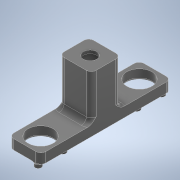
# Autodesk Inventor part: PotHolder
Saved by Autodesk Inventor 2022 (Build 260153000, 153)
## iProperties
Created: 2021-11-22
Part Number: PotHolder
Material: Genérico
Document SubType Name: Modeling
Designer: JK
Density: 1 g/cm^3
Appearance: Suave - Negro
Author: JK
Autodesk Inventor part; units mm, degrees
ref_plane "YZ Plane" through (0, 0, 0) normal (1, 0, 0) x (0, 1, 0)
ref_plane "XZ Plane" through (0, 0, 0) normal (0, 1, 0) x (-1, 0, 0)
ref_plane "XY Plane" through (0, 0, 0) normal (0, 0, 1) x (1, 0, 0)
sketch "Boceto7" plane through (0, 0, 0) normal (0, 1, 0) x (-1, 0, 0)
  line L0 (-6.5, 12.2) -> (6.5, 12.2)
  line L1 (6.5, 12.2) -> (6.5, -12.2)
  line L2 (6.5, -12.2) -> (-6.5, -12.2)
  line L3 (-6.5, -12.2) -> (-6.5, 12.2)
  line L4 (-6.5, 12.2) -> (6.5, -12.2) construction
  line L5 (6.5, 12.2) -> (-6.5, -12.2) construction
  line L6 (6.5, 12.2) -> (-6.5, 12.2)
  line L7 (-6.5, 12.2) -> (-6.5, 26.4)
  line L8 (-6.5, 26.4) -> (6.5, 26.4)
  line L9 (6.5, 26.4) -> (6.5, 12.2)
  line L10 (6.5, -12.2) -> (-6.5, -12.2)
  line L11 (-6.5, -12.2) -> (-6.5, -26.4)
  line L12 (-6.5, -26.4) -> (6.5, -26.4)
  line L13 (6.5, -26.4) -> (6.5, -12.2)
  line L14 (4.8, 24.8) -> (-4.8, 24.8)
  line L15 (-4.8, 24.8) -> (-4.8, 15.2)
  line L16 (-4.8, 15.2) -> (4.8, 15.2)
  line L17 (4.8, 15.2) -> (4.8, 24.8)
  line L18 (4.8, -15.2) -> (-4.8, -15.2)
  line L19 (-4.8, -15.2) -> (-4.8, -24.8)
  line L20 (-4.8, -24.8) -> (4.8, -24.8)
  line L21 (4.8, -24.8) -> (4.8, -15.2)
  line L22 (-4.8, 24.8) -> (4.8, 24.8)
  line L23 (4.8, 24.8) -> (4.8, 15.2)
  line L24 (4.8, 15.2) -> (-4.8, 15.2)
  line L25 (-4.8, 15.2) -> (-4.8, 24.8)
  line L26 (-4.8, 24.8) -> (4.8, 15.2) construction
  line L27 (4.8, 24.8) -> (-4.8, 15.2) construction
  line L28 (-4.8, -15.2) -> (4.8, -15.2)
  line L29 (4.8, -15.2) -> (4.8, -24.8)
  line L30 (4.8, -24.8) -> (-4.8, -24.8)
  line L31 (-4.8, -24.8) -> (-4.8, -15.2)
  line L32 (-4.8, -15.2) -> (4.8, -24.8) construction
  line L33 (4.8, -15.2) -> (-4.8, -24.8) construction
  point P0 (0, 0)
  point P1 (-6.5, 12.2)
  point P2 (0, 20)
  point P3 (0, -20)
  point P4 (0, -20)
  point P5 (0, 0)
  dimension "d23" = 9.6
  dimension "d24" = 9.6
  dimension "d26" = 1.6
  dimension "d28" = 3
  dimension "d30" = 1.6
  dimension "d31" = 3
  dimension "d43" = 40
  dimension "d48" = 13
  constraints: 68 end point, 14 parallel, 8 midpoint, 7 horizontal, 7 perpendicular, 6 collinear, 2 equal length, 1 point on line, 1 vertical alignment
  measures "d23" distance of L16.end L14.start
  measures "d24" distance of L15.end L16.end
  measures "d26" distance between parallel lines of L14 L8
  measures "d28" distance between parallel lines of L0 L16
  measures "d30" distance between parallel lines of L12 L20
  measures "d31" distance between parallel lines of L2 L18
  measures "d43" distance of point (0, -20) point (0, 20)
  measures "d48" distance between parallel lines of L7 L9
extrude "Extrusión4" add sketch "Boceto7" along normal blind 4
sketch "Boceto8" plane through (0, 4, 0) normal (0, 1, 0) x (1, 0, 0)
  circle A0 centre (0, -4.8061) radius 1.7
  circle A1 centre (0, 5.1939) radius 1.7
  point P0 (0, 0.1939)
  dimension "d35" = 3.4
  dimension "d49" = 5
  dimension "d50" = 5
  constraints: 2 centre point, 2 vertical alignment, 1 equal radius
  measures "d35" diameter of A0
  measures "d49" distance of A0.centre point (0, 0.194)
  measures "d50" distance of point (0, 0.194) A1.centre
fillet "Empalme3" radius 2 4 edges at (-6.5, 2, 26.4) (6.5, 2, 26.4) (-6.5, 2, -26.4) (6.5, 2, -26.4)
sketch "Boceto9" plane through (0, 4, 0) normal (0, 1, 0) x (1, 0, 0)
  line L0 (-6.5, 24.4) -> (-6.5, -24.4) projected
  line L1 (6.5, -6) -> (-6.5, -6)
  line L2 (-6.5, -6) -> (-6.5, 6)
  line L3 (-6.5, 6) -> (6.5, 6)
  line L4 (6.5, 6) -> (6.5, -6)
  line L5 (6.5, -6) -> (-6.5, 6) construction
  line L6 (-6.5, -6) -> (6.5, 6) construction
  arc A0 (6.5, 24.4) -> (4.5, 26.4) centre (4.5, 24.4) ccw projected
  line L7 (4.5, 26.4) -> (-4.5, 26.4) projected
  arc A1 (-4.5, 26.4) -> (-6.5, 24.4) centre (-4.5, 24.4) ccw projected
  line L8 (-6.5, 24.4) -> (-6.5, -24.4) projected
  arc A2 (-6.5, -24.4) -> (-4.5, -26.4) centre (-4.5, -24.4) ccw projected
  line L9 (-4.5, -26.4) -> (4.5, -26.4) projected
  arc A3 (4.5, -26.4) -> (6.5, -24.4) centre (4.5, -24.4) ccw projected
  line L10 (6.5, -24.4) -> (6.5, 24.4) projected
  line L11 (-4.8, -24.8) -> (-4.8, -15.2) projected
  line L12 (-4.8, -15.2) -> (4.8, -15.2) projected
  line L13 (4.8, -15.2) -> (4.8, -24.8) projected
  line L14 (4.8, -24.8) -> (-4.8, -24.8) projected
  line L15 (-4.8, 15.2) -> (-4.8, 24.8) projected
  line L16 (-4.8, 24.8) -> (4.8, 24.8) projected
  line L17 (4.8, 24.8) -> (4.8, 15.2) projected
  line L18 (4.8, 15.2) -> (-4.8, 15.2) projected
  point P0 (0, 0)
  dimension "d44" = 12
  constraints: 12 end point, 2 midpoint, 2 parallel, 1 horizontal, 1 perpendicular, 1 point on line
  measures "d44" distance between parallel lines of L3 L1
extrude "Extrusión6" add sketch "Boceto9" along normal blind 18.3 contours L3 L4 L1 L0
fillet "Empalme4" radius 2 6 edges at (6.5, 13.15, 6) (6.5, 13.15, -6) (-6.5, 13.15, -6) (-6.5, 13.15, 6) (0, 4, -6) (0, 4, 6)
sketch "Boceto11" plane through (0, 0, 0) normal (0, -1, 0) x (1, 0, 0)
  circle A0 centre (0, 20) radius 5.1
  line L0 (-4.8, 15.2) -> (4.8, 15.2) projected
  line L1 (-4.8, 24.8) -> (4.8, 24.8)
  line L2 (4.8, 24.8) -> (4.8, 15.2)
  line L3 (4.8, 15.2) -> (-4.8, 15.2)
  line L4 (-4.8, 15.2) -> (-4.8, 24.8)
  line L5 (-4.8, 24.8) -> (4.8, 15.2) construction
  line L6 (4.8, 24.8) -> (-4.8, 15.2) construction
  line L7 (4.8, -24.8) -> (4.8, -15.2) projected
  line L8 (-4.8, -15.2) -> (4.8, -15.2)
  line L9 (4.8, -15.2) -> (4.8, -24.8)
  line L10 (4.8, -24.8) -> (-4.8, -24.8)
  line L11 (-4.8, -24.8) -> (-4.8, -15.2)
  line L12 (-4.8, -15.2) -> (4.8, -24.8) construction
  line L13 (4.8, -15.2) -> (-4.8, -24.8) construction
  circle A1 centre (0, -20) radius 5.1
  point P0 (0, 0)
  point P1 (0, 20)
  point P2 (0, 20)
  dimension "d54" = 10.2
  dimension "d55" = 10.2
  constraints: 24 end point, 5 midpoint, 4 parallel, 2 centre point, 2 coincident, 2 horizontal, 2 perpendicular
  measures "d54" diameter of A0
  measures "d55" diameter of A1
extrude "Extrusión8" cut sketch "Boceto11" against normal through all contours A0 L2 | L2 A0 L0 L4 L1 | L1 A0 | A0 L0 | L4 A0 | A1 L10 L11 L8 L7 | L7 A1 | A1 L10 | L8 A1 | A1 L11
sketch "Boceto12" plane through (0, 0, 0) normal (0, -1, 0) x (1, 0, 0)
  arc A0 (4.8, 18.2766) -> (4.8, 21.7234) centre (0, 20) ccw projected
  circle A1 centre (0, 20) radius 5.1
  arc A2 (4.8, -21.7234) -> (4.8, -18.2766) centre (0, -20) ccw projected
  circle A3 centre (0, -20) radius 5.1
  arc A4 (1.7234, -15.2) -> (-1.7234, -15.2) centre (0, -20) ccw projected
  line L0 (4.8, -15.2) -> (1.7234, -15.2) projected
  line L1 (4.8, -18.2766) -> (4.8, -15.2) projected
  arc A5 (4.8, -21.7234) -> (4.8, -18.2766) centre (0, -20) ccw projected
  line L2 (4.8, -24.8) -> (4.8, -21.7234) projected
  line L3 (1.7234, -24.8) -> (4.8, -24.8) projected
  arc A6 (-1.7234, -24.8) -> (1.7234, -24.8) centre (0, -20) ccw projected
  line L4 (-4.8, -24.8) -> (-1.7234, -24.8) projected
  line L5 (-4.8, -21.7234) -> (-4.8, -24.8) projected
  arc A7 (-4.8, -18.2766) -> (-4.8, -21.7234) centre (0, -20) ccw projected
  line L6 (-4.8, -15.2) -> (-4.8, -18.2766) projected
  line L7 (-1.7234, -15.2) -> (-4.8, -15.2) projected
  arc A8 (1.7234, 24.8) -> (-1.7234, 24.8) centre (0, 20) ccw projected
  line L8 (4.8, 24.8) -> (1.7234, 24.8) projected
  line L9 (4.8, 21.7234) -> (4.8, 24.8) projected
  arc A9 (4.8, 18.2766) -> (4.8, 21.7234) centre (0, 20) ccw projected
  line L10 (4.8, 15.2) -> (4.8, 18.2766) projected
  line L11 (1.7234, 15.2) -> (4.8, 15.2) projected
  arc A10 (-1.7234, 15.2) -> (1.7234, 15.2) centre (0, 20) ccw projected
  line L12 (-4.8, 15.2) -> (-1.7234, 15.2) projected
  line L13 (-4.8, 18.2766) -> (-4.8, 15.2) projected
  arc A11 (-4.8, 21.7234) -> (-4.8, 18.2766) centre (0, 20) ccw projected
  line L14 (-4.8, 24.8) -> (-4.8, 21.7234) projected
  line L15 (-1.7234, 24.8) -> (-4.8, 24.8) projected
  arc A12 (4.5, -26.4) -> (6.5, -24.4) centre (4.5, -24.4) ccw projected
  line L16 (6.5, 24.4) -> (6.5, -24.4) projected
  arc A13 (6.5, 24.4) -> (4.5, 26.4) centre (4.5, 24.4) ccw projected
  line L17 (-4.5, 26.4) -> (4.5, 26.4) projected
  arc A14 (-4.5, 26.4) -> (-6.5, 24.4) centre (-4.5, 24.4) ccw projected
  line L18 (-6.5, -24.4) -> (-6.5, 24.4) projected
  arc A15 (-6.5, -24.4) -> (-4.5, -26.4) centre (-4.5, -24.4) ccw projected
  line L19 (4.5, -26.4) -> (-4.5, -26.4) projected
  point P0 (0, 0)
  point P1 (-1.7234, 24.8)
  point P2 (-4.8, 21.7234)
  point P3 (1.7234, 24.8)
  point P4 (4.8, 18.2766)
  point P5 (-1.7234, 15.2)
  point P6 (-1.7234, -15.2)
  point P7 (-4.8, -18.2766)
  point P8 (-1.7234, -24.8)
  point P9 (4.8, -21.7234)
  point P10 (1.7234, -15.2)
  constraints: 2 centre point, 2 coincident
extrude "Extrusión9" add sketch "Boceto12" against normal up to surface (4 mm away) contours L10 L11 A1 | A1 L8 L9 | L12 L13 A1 | A1 L14 L15 | L2 L3 A3 | A3 L0 L1 | L4 L5 A3 | A3 L6 L7
fillet "Empalme5" radius 0.75 16 edges at (-5.1, 0, 20) (0, 0, 14.9) (5.1, 0, 20) (0, 0, 25.1) (-3.6062, 0, 23.6062) (-3.6062, 0, 16.3938) (3.6062, 0, 16.3938) (3.6062, 0, 23.6062) (-5.1, 0, -20) (0, 0, -25.1) (5.1, 0, -20) (0, 0, -14.9) (-3.6062, 0, -16.3938) (-3.6062, 0, -23.6062) (3.6062, 0, -23.6062) (3.6062, 0, -16.3938)
sketch "Boceto14" plane through (0, 0, 0) normal (0, -1, 0) x (1, 0, 0)
  circle A0 centre (0, 20) radius 5.85 projected
  arc A1 (6.5, -24.4) -> (4.5, -26.4) centre (4.5, -24.4) ccw projected
  line L0 (6.5, 24.4) -> (6.5, -24.4) projected
  arc A2 (4.5, 26.4) -> (6.5, 24.4) centre (4.5, 24.4) ccw projected
  line L1 (-4.5, 26.4) -> (4.5, 26.4) projected
  arc A3 (-6.5, 24.4) -> (-4.5, 26.4) centre (-4.5, 24.4) ccw projected
  line L2 (-6.5, -24.4) -> (-6.5, 24.4) projected
  arc A4 (-4.5, -26.4) -> (-6.5, -24.4) centre (-4.5, -24.4) ccw projected
  line L3 (4.5, -26.4) -> (-4.5, -26.4) projected
  circle A5 centre (0, -20) radius 5.1531
  circle A6 centre (4, -25) radius 1.25
  circle A7 centre (4, -15) radius 1.25
  point P0 (0, 0)
  dimension "d65" = 2.5
  dimension "d66" = 4
  dimension "d72" = 5
  dimension "d73" = 5
  constraints: 8 centre point, 1 equal radius, 1 tangent, 1 vertical alignment
  measures "d65" diameter of A7
  measures "d66" horizontal distance of A5.centre A7.centre
  measures "d72" vertical distance of A7.centre A5.centre
  measures "d73" vertical distance of A6.centre A5.centre
extrude "Extrusión11" add sketch "Boceto14" along normal blind 2 and the other way blind 1 contours A7 | A6 A1 | A1 A6
mirror "Simetría1" about plane through (0, 0, 0) normal (0, 0, 1) of "Extrusión11"
fillet "Empalme7" radius 0.75 16 edges at (3.6813, 0.2573, 16.2087) (2.7913, 0.1153, 15.3185) (5.0236, 0, 15.7175) (4.0791, 0, 13.7525) (2.7913, 0.1153, 24.6815) (3.6813, 0.2573, 23.7913) (4.0791, 0, 26.2475) (5.0236, 0, 24.2825) (2.7913, 0.1153, -15.3185) (3.6813, 0.2573, -16.2087) (4.0791, 0, -13.7525) (5.0236, 0, -15.7175) (2.7913, 0.1153, -24.6815) (3.6813, 0.2573, -23.7913) (4.0791, 0, -26.2475) (5.0236, 0, -24.2825)
sketch "Boceto16" plane through (0, 22.3, 0) normal (0, 1, 0) x (1, 0, 0)
  circle A0 centre (0, 0) radius 2.7
  dimension "d77" = 5.4
  constraints: 1 centre point, 1 coincident
  measures "d77" diameter of A0
extrude "Extrusión13" cut sketch "Boceto16" against normal through all
sketch "Boceto17" plane through (0, 0, 0) normal (0, -1, 0) x (1, 0, 0)
  circle A0 centre (0, 0) radius 4.6
  dimension "d80" = 9.2
  constraints: 1 centre point, 1 coincident
  measures "d80" diameter of A0
extrude "Extrusión14" cut sketch "Boceto17" against normal blind 21
fillet "Empalme8" radius 1 1 edges at (-4.6, 0, 0)
sketch "Boceto15" plane through (0, 0, 0) normal (0, -1, 0) x (1, 0, 0)
  line L0 (6.5, 24.4) -> (6.5, -24.4) projected
  line L1 (-6.5, 29.6309) -> (6.5, 29.6309)
  line L2 (6.5, 29.6309) -> (6.5, 10.3691)
  line L3 (6.5, 10.3691) -> (-6.5, 10.3691)
  line L4 (-6.5, 10.3691) -> (-6.5, 29.6309)
  arc A0 (4.891, 16.7906) -> (4.891, 23.2094) centre (0, 20) ccw projected
  line L5 (-6.5, 29.6309) -> (6.5, 10.3691) construction
  line L6 (6.5, 29.6309) -> (-6.5, 10.3691) construction
  line L7 (13.0536, 10.3534) -> (-14.653, 10.3534)
  line L8 (-14.653, 10.3534) -> (-14.653, -30.0958)
  line L9 (-14.653, -30.0958) -> (13.0536, -30.0958)
  line L10 (13.0536, -30.0958) -> (13.0536, 10.3534)
  point P0 (0, 0)
  point P1 (3.6743, 15.4478)
  point P2 (3.6743, 24.5522)
  point P3 (8, 10.3534)
  point P4 (-8, 10.3534)
  constraints: 20 end point, 4 parallel, 2 horizontal, 2 midpoint, 2 perpendicular, 1 point on line
sketch "Boceto10" plane through (0, 0, 0) normal (0, -1, 0) x (1, 0, 0)
  line L0 (8, 25.8) -> (8, 10.3534) projected
  arc A0 (8, 25.8) -> (6, 27.8) centre (6, 25.8) ccw projected
  line L1 (-6, 27.8) -> (6, 27.8) projected
  arc A1 (-6, 27.8) -> (-8, 25.8) centre (-6, 25.8) ccw projected
  line L2 (-8, 10.3534) -> (-8, 25.8) projected
  line L3 (-4.8, 15.2) -> (4.8, 15.2) projected
  line L4 (-2.4608, 24.8) -> (2.8, 24.8)
  line L5 (2.8, 24.8) -> (2.8, 15.2)
  line L6 (2.8, 15.2) -> (-2.4608, 15.2)
  line L7 (-2.4608, 15.2) -> (-2.4608, 24.8)
  line L8 (-2.4608, 24.8) -> (2.8, 15.2) construction
  line L9 (2.8, 24.8) -> (-2.4608, 15.2) construction
  line L10 (-4.8, -24.8) -> (4.8, -24.8) projected
  line L11 (-2.6635, -15.2) -> (2.8, -15.2)
  line L12 (2.8, -15.2) -> (2.8, -24.8)
  line L13 (2.8, -24.8) -> (-2.6635, -24.8)
  line L14 (-2.6635, -24.8) -> (-2.6635, -15.2)
  line L15 (-2.6635, -15.2) -> (2.8, -24.8) construction
  line L16 (2.8, -15.2) -> (-2.6635, -24.8) construction
  line L17 (-8, 10.3534) -> (8, 10.3534) projected
  point P0 (0, 0)
  point P1 (0.1696, 20)
  point P2 (0.0682, -20)
  constraints: 24 end point, 4 midpoint, 4 parallel, 2 horizontal, 2 perpendicular, 2 point on line, 1 collinear
